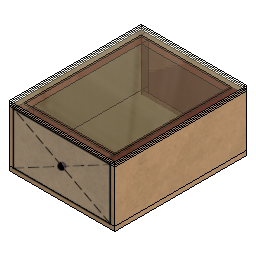
valkyrie Drybox obssesion paramectric_v15 (Autodesk Fusion 360 design; units mm, degrees)
Autodesk Fusion 360 part; units mm, degrees
sketch "Sketch2" plane through (0, 0, 0) normal (0, 0, 1) x (1, 0, 0) in component "Base "
  line L0 (201.5693, 10.5193) -> (481.5693, 10.5193)
  line L1 (481.5693, 10.5193) -> (481.5693, 360.5193)
  line L2 (481.5693, 360.5193) -> (201.5693, 360.5193)
  line L3 (201.5693, 360.5193) -> (201.5693, 10.5193)
  dimension "d38" = 280
  dimension "d39" = 350
  constraint horizontal L0
  constraint vertical L1
  constraint horizontal L2
  constraint vertical L3
  measures "d38" distance of L0.start L0.end
  measures "d39" distance of L0.start L2.end
extrude "Extrude2" add sketch "Sketch2" along normal blind 12 makes body 1 in component "Base "
sketch "Sketch1" plane through (0, 0, 0) normal (0, 1, 0) x (1, 0, 0) in component "Bow"
  line L0 (128, 68) -> (-128, 68)
  line L1 (-128, 68) -> (-128, -68)
  line L2 (-128, -68) -> (128, -68)
  line L3 (128, -68) -> (128, 68)
  line L4 (128, 68) -> (-128, -68) construction
  line L5 (-128, 68) -> (128, -68) construction
  dimension "d1" = 256
  dimension "d6" = 136
  constraint horizontal L0
  constraint perpendicular L0 L1
  constraint parallel L0 L2
  constraint parallel L1 L3
  constraint coincident L4 origin
  constraint coincident L5 origin
  measures "d1" distance of L1.end L2.end
  measures "d6" distance of L0.end L1.end
extrude "Extrude1" add sketch "Sketch1" along normal blind 12 separate body makes body 2 in component "Bow"
sketch "Sketch1 (2)" plane through (268, 0, 80) normal (1, 0, 0) x (0, 1, 0) in component "starboardt Side"
  line L0 (0, 68) -> (0, -68)
  line L1 (0, -68) -> (12, -68)
  line L2 (12, -68) -> (12, 68)
  line L3 (12, 68) -> (0, 68)
  line L4 (12, 68) -> (362, 68)
  line L5 (362, 68) -> (362, -68)
  line L6 (362, -68) -> (12, -68)
  line L7 (12, -68) -> (12, 68)
  dimension "d9" = 350
  dimension "d10" = 136
  constraint horizontal L4
  constraint vertical L5
  constraint horizontal L6
  constraint vertical L7
  constraint coincident L2.end L3.start
  measures "d9" distance of L2.end L4.end
  measures "d10" distance of L2.end L1.end
extrude "Extrude1'" add sketch "Sketch1 (2)" against normal blind 12 separate body contours L2 L4 L5 L6 L7 makes body 3 in component "starboardt Side"
sketch "Sketch1 (3)" plane through (12, 0, 80) normal (-1, 0, 0) x (0, -1, 0) in component "Port side"
  line L0 (0, -68) -> (0, 68)
  line L1 (0, 68) -> (-12, 68)
  line L2 (-12, 68) -> (-12, -68)
  line L3 (-12, -68) -> (0, -68)
  line L4 (-12, 68) -> (-362, 68)
  line L5 (-362, 68) -> (-362, -68)
  line L6 (-362, -68) -> (-12, -68)
  line L7 (-12, -68) -> (-12, 68)
  dimension "d13" = 350
  dimension "d14" = 136
  constraint horizontal L4
  constraint vertical L5
  constraint horizontal L6
  constraint vertical L7
  constraint coincident L1.end L2.start
  measures "d13" distance of L1.end L4.end
  measures "d14" distance of L1.end L2.end
extrude "Extrude1''" add sketch "Sketch1 (3)" against normal blind 12 separate body contours L2 L4 L5 L6 L7 makes body 4 in component "Port side"
sketch "Sketch1 (4)" plane through (12, 350, 0) normal (0, 1, 0) x (-1, 0, 0) in component "Stern"
  line L0 (-268, 148) -> (-268, 12)
  line L1 (-268, 12) -> (-256, 12)
  line L2 (-256, 12) -> (-256, 148)
  line L3 (-256, 148) -> (-268, 148)
  line L4 (-256, 148) -> (0, 148)
  line L5 (0, 148) -> (0, 12)
  line L6 (0, 12) -> (-256, 12)
  line L7 (-256, 12) -> (-256, 148)
  dimension "d20" = 136
  dimension "d21" = 256
  constraint coincident L2.end L3.start
  constraint vertical L7
  constraint horizontal L4
  constraint vertical L5
  constraint horizontal L6
  measures "d20" distance of L2.end L1.end
  measures "d21" distance of L2.end L4.end
extrude "Extrude1'''" add sketch "Sketch1 (4)" against normal blind 12 separate body contours L2 L4 L5 L6 L7 makes body 5 in component "Stern"
sketch "Sketch1 (5)" plane through (268, 0, 0) normal (-1, 0, 0) x (0, -1, 0) in component "insulation Starboard side"
  line L0 (-350, 12) -> (0, 12)
  line L1 (0, 12) -> (0, 148)
  line L2 (0, 148) -> (-350, 148)
  line L3 (-350, 148) -> (-350, 12)
  line L4 (-288, 156.4658) -> (38, 156.4658)
  line L5 (38, 156.4658) -> (38, 20.4658)
  line L6 (38, 20.4658) -> (-288, 20.4658)
  line L7 (-288, 20.4658) -> (-288, 156.4658)
  dimension "d46" = 136
  dimension "d47" = 326
  constraint horizontal L4
  constraint vertical L5
  constraint horizontal L6
  constraint vertical L7
  measures "d46" distance of L4.start L6.end
  measures "d47" distance of L4.start L4.end
extrude "Extrude1''''" add sketch "Sketch1 (5)" along normal blind 20 separate body contours L1 L2 L6 L7 | L1 L2 L4 L5 L6 L7 makes body 6 in component "insulation Starboard side"
sketch "Sketch1 (6)" plane through (12, 0, 0) normal (1, 0, 0) x (0, 1, 0) in component "insulation Port side"
  line L0 (0, 148) -> (0, 12)
  line L1 (0, 12) -> (350, 12)
  line L2 (350, 12) -> (350, 148)
  line L3 (350, 148) -> (0, 148)
  line L4 (18.8584, 118.8317) -> (344.8584, 118.8317)
  line L5 (344.8584, 118.8317) -> (344.8584, -17.1683)
  line L6 (344.8584, -17.1683) -> (18.8584, -17.1683)
  line L7 (18.8584, -17.1683) -> (18.8584, 118.8317)
  dimension "d55" = 326
  dimension "d56" = 136
  constraint horizontal L4
  constraint vertical L5
  constraint horizontal L6
  constraint vertical L7
  measures "d55" distance of L4.start L4.end
  measures "d56" distance of L4.start L6.end
extrude "Extrude1'''''" add sketch "Sketch1 (6)" along normal blind 20 separate body contours L1 L4 L5 L7 makes body 7 in component "insulation Port side"
sketch "Sketch1 (7)" plane through (140, 12, 80) normal (0, 1, 0) x (-1, 0, 0) in component "insulation Bow"
  line L0 (-128, 68) -> (-128, -68)
  line L1 (-128, -68) -> (128, -68)
  line L2 (128, -68) -> (128, 68)
  line L3 (128, 68) -> (-128, 68)
  line L4 (-130.6712, 134.0558) -> (85.3288, 134.0558)
  line L5 (85.3288, 134.0558) -> (85.3288, -1.9442)
  line L6 (85.3288, -1.9442) -> (-130.6712, -1.9442)
  line L7 (-130.6712, -1.9442) -> (-130.6712, 134.0558)
  dimension "d63" = 216
  dimension "d64" = 136
  constraint horizontal L4
  constraint vertical L5
  constraint horizontal L6
  constraint vertical L7
  measures "d63" distance of L4.start L4.end
  measures "d64" distance of L4.start L6.end
extrude "Extrude1''''''" add sketch "Sketch1 (7)" along normal blind 20 separate body contours L0 L3 L5 L6 | L0 L3 L4 L5 L6 L7 makes body 8 in component "insulation Bow"
sketch "Sketch1 (8)" plane through (-12, 338, 0) normal (0, -1, 0) x (1, 0, 0) in component "insulation Stern"
  line L0 (24, 12) -> (280, 12)
  line L1 (280, 12) -> (280, 148)
  line L2 (280, 148) -> (24, 148)
  line L3 (24, 148) -> (24, 12)
  line L4 (-124.9936, 135.96) -> (91.0064, 135.96)
  line L5 (91.0064, 135.96) -> (91.0064, -0.04)
  line L6 (91.0064, -0.04) -> (-124.9936, -0.04)
  line L7 (-124.9936, -0.04) -> (-124.9936, 135.96)
  dimension "d71" = 216
  dimension "d72" = 136
  constraint horizontal L4
  constraint vertical L5
  constraint horizontal L6
  constraint vertical L7
  measures "d71" distance of L4.start L4.end
  measures "d72" distance of L4.start L6.end
extrude "Extrude1'''''''" add sketch "Sketch1 (8)" along normal blind 20 separate body contours L0 L3 L4 L5 | L0 L3 L4 L5 L6 L7 makes body 9 in component "insulation Stern"
sketch "Sketch1 (9)" plane through (138, -12, 0) normal (0, 0, -1) x (1, 0, 0) in component "insulation base"
  line L0 (-138, -12) -> (-138, -362)
  line L1 (-138, -362) -> (142, -362)
  line L2 (142, -362) -> (142, -12)
  line L3 (142, -12) -> (-138, -12)
  line L4 (-377.3205, -251.0817) -> (-129.3205, -251.0817)
  line L5 (-129.3205, -251.0817) -> (-129.3205, 66.9183)
  line L6 (-129.3205, 66.9183) -> (-377.3205, 66.9183)
  line L7 (-377.3205, 66.9183) -> (-377.3205, -251.0817)
  dimension "d79" = 248
  dimension "d80" = 318
  constraint horizontal L4
  constraint vertical L5
  constraint horizontal L6
  constraint vertical L7
  measures "d79" distance of L4.start L4.end
  measures "d80" distance of L4.start L6.end
extrude "Extrude1''''''''" add sketch "Sketch1 (9)" along normal blind 20 separate body contours L0 L3 L4 L5 | L0 L3 L4 L5 L6 L7 makes body 10 in component "insulation base"
sketch "Sketch1 (10)" plane through (-12, -20.5212, 148) normal (0, 0, 1) x (-1, 0, 0) in component "Lid inner"
  line L0 (0, -358.5212) -> (-280, -358.5212)
  line L1 (-280, -358.5212) -> (-280, -8.5212)
  line L2 (-280, -8.5212) -> (0, -8.5212)
  line L3 (0, -8.5212) -> (0, -358.5212)
  line L4 (-12, -370.5212) -> (-12, -20.5212)
  line L5 (-12, -20.5212) -> (-24, -20.5212)
  line L6 (-24, -20.5212) -> (-24, -370.5212)
  line L7 (-24, -370.5212) -> (-12, -370.5212)
  point P0 (0, -358.5212)
  point P1 (-280, -8.5212)
  constraint horizontal L0
  constraint vertical L1
  constraint horizontal L2
  constraint vertical L3
  constraint coincident P1 L1.end
  constraint coincident P0 L0.start
extrude "Extrude1'''''''''" add sketch "Sketch1 (10)" along normal blind 4 separate body contours L0 L1 L2 L3 L4 L5 L6 | L0 L4 L5 L6 makes body 11 in component "Lid inner"
sketch "Sketch1 (11)" plane through (12, 12, 152) normal (0, 0, 1) x (-1, 0, 0) in component "spacers"
  line L0 (12, 12) -> (-268, 12)
  line L1 (-268, 12) -> (-268, -338)
  line L2 (-268, -338) -> (12, -338)
  line L3 (12, -338) -> (12, 12)
  line L4 (12, -338) -> (-8, -338)
  line L5 (-8, -338) -> (-8, 12)
  line L6 (-8, 12) -> (12, 12)
  line L7 (12, 12) -> (12, -338)
  line L8 (-268, -338) -> (-248, -338)
  line L9 (-248, -338) -> (-248, 12)
  line L10 (-248, 12) -> (-268, 12)
  line L11 (-268, 12) -> (-268, -338)
  line L12 (-8, -338) -> (-248, -338)
  line L13 (-248, -338) -> (-248, -318)
  line L14 (-248, -318) -> (-8, -318)
  line L15 (-8, -318) -> (-8, -338)
  line L16 (-8, 12) -> (-248, 12)
  line L17 (-248, 12) -> (-248, -8)
  line L18 (-248, -8) -> (-8, -8)
  line L19 (-8, -8) -> (-8, 12)
  line L20 (0, 12) -> (-256, 12)
  dimension "d217" = 20
  dimension "d218" = 20
  dimension "d219" = 240
  dimension "d220" = 20
  dimension "d221" = 20
  constraint horizontal L4
  constraint vertical L5
  constraint horizontal L6
  constraint vertical L7
  constraint coincident L0 L5.end
  constraint coincident L2.end L3.start
  constraint horizontal L8
  constraint vertical L9
  constraint horizontal L10
  constraint vertical L11
  constraint coincident L1.end L2.start
  constraint horizontal L12
  constraint vertical L13
  constraint horizontal L14
  constraint vertical L15
  constraint horizontal L16
  constraint vertical L17
  constraint horizontal L18
  constraint vertical L19
  constraint collinear L10 L20
  constraint collinear L9 L17
  measures "d217" distance of L2.end L4.end
  measures "d218" distance of L1.end L8.end
  measures "d219" distance of L4.end L8.end
  measures "d220" distance of L4.end L14.end
  measures "d221" distance of L5.end L18.end
extrude "Extrude1''''''''''" add sketch "Sketch1 (11)" along normal blind 4 separate body contours L0 L5 L9 L16 L17 L18 L19 L20 | L2 L5 L9 L12 L13 L14 L15 makes body 12 at (100, 343.3333, 152) makes body 13 at (180, 13.3333, 152) in component "spacers"
extrude "Extrude2'" add sketch "Sketch1 (11)" along normal blind 4 contours L0 L2 L3 L4 L5 L6 L7 L15 L19 L20 | L0 L1 L2 L8 L9 L10 L11 L13 L17 L20 bodies 12 13 in component "spacers"
sketch "Sketch1 (12)" plane through (0, 0, 152) normal (0, 0, 1) x (-1, 0, 0) in component "lid Outer"
  line L0 (-280, 0) -> (0, 0)
  line L1 (0, 0) -> (0, -350)
  line L2 (0, -350) -> (-280, -350)
  line L3 (-280, -350) -> (-280, 0)
  point P0 (-280, 0)
  point P1 (0, -350)
  constraint horizontal L0
  constraint vertical L1
  constraint horizontal L2
  constraint vertical L3
  constraint coincident P1 L1.end
  constraint coincident P0 L0.start
extrude "Extrude1'''''''''''" add sketch "Sketch1 (12)" along normal blind 4 separate body makes body 14 in component "lid Outer"
imported_body "Base Feature1" makes body 15 makes body 16 makes body 17 makes body 18 makes body 19 makes body 20 makes body 21 makes body 22 in component "11435A13_Steel Drawer Slides"
imported_body "Base Feature1'" makes body 23 makes body 24 makes body 25 makes body 26 makes body 27 makes body 28 makes body 29 makes body 30 in component "11435A13_Steel Drawer Slides (1)"
component "Base " placed x (1, 0, 0) y (0, 1, 0) z (0, 0, 1) at (-201.5693, -10.5193, 0)
component "Bow" placed x (1, 0, 0) y (0, 1, 0) z (0, 0, 1) at (140, 0, 80)
component "starboardt Side" placed x (1, 0, 0) y (0, 1, 0) z (0, 0, 1) at (12, -12, 0)
component "Port side" placed x (1, 0, 0) y (0, 1, 0) z (0, 0, 1) at (-12, -12, 0)
component "Stern" placed x (1, 0, 0) y (0, 1, 0) z (0, 0, 1) at (0, 0, 0)
component "insulation Starboard side" placed x (1, 0, 0) y (0, 1, 0) z (0, 0, 1) at (0, 50, -8.4658)
component "insulation Port side" placed x (1, 0, 0) y (0, 1, 0) z (0, 0, 1) at (0, -6.8584, 29.1683)
component "insulation Bow" placed x (1, 0, 0) y (0, 1, 0) z (0, 0, 1) at (-22.6712, 0, -66.0558)
component "insulation Stern" placed x (1, 0, 0) y (0, 1, 0) z (0, 0, 1) at (168.9936, 0, 12.04)
component "insulation base" placed x (1, 0, 0) y (0, 1, 0) z (0, 0, 1) at (251.3205, 90.9183, 32)
component "Lid" placed x (1, 0, 0) y (0, 1, 0) z (0, 0, 1) at (0, 0, 0)
component "Lid inner" placed x (1, 0, 0) y (0, 1, 0) z (0, 0, 1) at (12, 12, 0) in component "Lid"
component "spacers" placed x (1, 0, 0) y (0, 1, 0) z (0, 0, 1) at (0, 0, 0) in component "Lid"
component "lid Outer" placed x (1, 0, 0) y (0, 1, 0) z (0, 0, 1) at (0, 0, 4) in component "Lid"
equation "d1 = drawerWidth - ( thicknessMDF * 2 )"
equation "drawerWidth = 280 mm"
equation "drawerHeight = 150 mm - 14 mm"
equation "drawerDepth = 350 mm"
equation "thicknessMDF = 12 mm"
equation "d6 = drawerHeight"
equation "d7 = thicknessMDF"
equation "d9 = drawerDepth"
equation "d10 = drawerHeight"
equation "d11 = -thicknessMDF"
equation "d13 = drawerDepth"
equation "d14 = drawerHeight"
equation "d15 = -thicknessMDF"
equation "d20 = drawerHeight"
equation "d21 = drawerWidth - ( thicknessMDF * 2 )"
equation "d22 = -thicknessMDF"
equation "d38 = drawerWidth"
equation "d39 = drawerDepth"
equation "d40 = thicknessMDF"
equation "d46 = drawerHeight"
equation "d47 = drawerDepth - ( 2 * thicknessMDF )"
equation "thicknessInsulation = 20 mm"
equation "d49 = thicknessInsulation"
equation "d55 = drawerDepth - ( 2 * thicknessMDF )"
equation "d56 = drawerHeight"
equation "d57 = thicknessInsulation"
equation "d63 = drawerWidth - ( 2 * thicknessMDF ) - ( 2 * thicknessInsulation )"
equation "d64 = drawerHeight"
equation "d65 = thicknessInsulation"
equation "d71 = drawerWidth - ( 2 * thicknessMDF ) - 2 * thicknessInsulation"
equation "d72 = drawerHeight"
equation "d73 = thicknessInsulation"
equation "d79 = drawerWidth - ( thicknessMDF ) - ( thicknessInsulation )"
equation "d80 = drawerDepth - ( thicknessMDF ) - ( thicknessInsulation )"
equation "d81 = thicknessInsulation"
equation "d200 = thicknessMDF"
equation "d208 = thicknessMDF"
equation "d212 = thicknessMDF"
equation "d213 = thicknessMDF"
